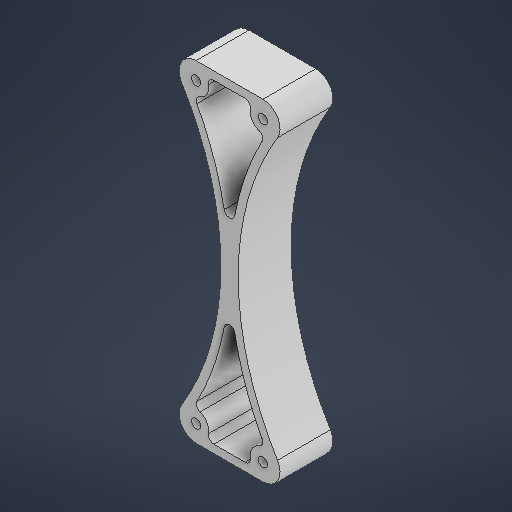
# Autodesk Inventor part: fan_connector_01
Saved by Autodesk Inventor 2026.2 (Build 302298010, 298A)
## iProperties
Created: 2026-05-14
Part Number: fan_connector_01
Material: 一般
Document SubType Name: Modeling
Designer: nyxeon
Density: 1 g/cm^3
Appearance: 既定
Author: nyxeon
Autodesk Inventor part; units mm, degrees
ref_plane "YZ Plane" through (0, 0, 0) normal (1, 0, 0) x (0, 1, 0)
ref_plane "XZ Plane" through (0, 0, 0) normal (0, 1, 0) x (-1, 0, 0)
ref_plane "XY Plane" through (0, 0, 0) normal (0, 0, 1) x (1, 0, 0)
sketch "スケッチ1" plane through (0, 0, 0) normal (0, 0, 1) x (1, 0, 0)
  line L0 (216.819241, 50.161956) -> (211.869241, 50.161956) construction
  line L1 (211.869241, 59.337068) -> (211.869241, 50.161956) construction
  arc A0 (211.869241, 59.337068) -> (211.361116, 60.6691) centre (209.869241, 59.337068) ccw construction
  line L2 (209.369241, 62.9) -> (211.361116, 60.6691) construction
  line L3 (209.369241, 63.9) -> (209.369241, 62.9) construction
  arc A1 (207.869241, 65.4) -> (209.369241, 63.9) centre (209.369241, 65.4) ccw construction
  line L4 (207.869241, 65.4) -> (207.869241, 85.3) construction
  arc A2 (207.869241, 85.3) -> (201.869241, 91.3) centre (201.869241, 85.3) ccw construction
  line L5 (201.869241, 91.3) -> (181.969241, 91.3) construction
  arc A3 (180.469241, 92.8) -> (181.969241, 91.3) centre (181.969241, 92.8) ccw construction
  line L6 (180.469241, 92.8) -> (179.469241, 92.8) construction
  line L7 (179.469241, 92.8) -> (177.238341, 94.791875) construction
  arc A4 (177.238341, 94.791875) -> (175.906309, 95.3) centre (175.906309, 93.3) ccw construction
  line L8 (175.906309, 95.3) -> (154.307286, 95.3) construction
  arc A5 (154.307286, 95.3) -> (137.927787, 100.25) centre (116.569241, 0) ccw construction
  line L9 (95.210695, 100.25) -> (137.927787, 100.25) construction
  arc A6 (95.210695, 100.25) -> (78.831197, 95.3) centre (116.569241, 0) ccw construction
  line L10 (57.232173, 95.3) -> (78.831197, 95.3) construction
  arc A7 (57.232173, 95.3) -> (55.900142, 94.791875) centre (57.232173, 93.3) ccw construction
  line L11 (53.669241, 92.8) -> (55.900142, 94.791875) construction
  line L12 (52.669241, 92.8) -> (53.669241, 92.8) construction
  arc A8 (51.169241, 91.3) -> (52.669241, 92.8) centre (51.169241, 92.8) ccw construction
  line L13 (31.269241, 91.3) -> (51.169241, 91.3) construction
  arc A9 (31.269241, 91.3) -> (25.269241, 85.3) centre (31.269241, 85.3) ccw construction
  line L14 (25.269241, 65.4) -> (25.269241, 85.3) construction
  arc A10 (23.769241, 63.9) -> (25.269241, 65.4) centre (23.769241, 65.4) ccw construction
  line L15 (23.769241, 63.9) -> (23.769241, 62.9) construction
  line L16 (23.769241, 62.9) -> (21.777366, 60.6691) construction
  arc A11 (21.777366, 60.6691) -> (21.269241, 59.337068) centre (23.269241, 59.337068) ccw construction
  line L17 (21.269241, 59.337068) -> (21.269241, 37.738044) construction
  arc A12 (21.269241, 37.738044) -> (16.319241, 21.358546) centre (116.569241, 0) ccw construction
  line L18 (16.319241, -21.358546) -> (16.319241, 21.358546) construction
  arc A13 (16.319241, -21.358546) -> (21.269241, -37.738044) centre (116.569241, 0) ccw construction
  line L19 (21.269241, -59.337068) -> (21.269241, -37.738044) construction
  arc A14 (21.269241, -59.337068) -> (21.777366, -60.6691) centre (23.269241, -59.337068) ccw construction
  line L20 (23.769241, -62.9) -> (21.777366, -60.6691) construction
  line L21 (23.769241, -63.9) -> (23.769241, -62.9) construction
  arc A15 (25.269241, -65.4) -> (23.769241, -63.9) centre (23.769241, -65.4) ccw construction
  line L22 (25.269241, -65.4) -> (25.269241, -85.3) construction
  arc A16 (25.269241, -85.3) -> (31.269241, -91.3) centre (31.269241, -85.3) ccw construction
  line L23 (31.269241, -91.3) -> (51.169241, -91.3) construction
  arc A17 (52.669241, -92.8) -> (51.169241, -91.3) centre (51.169241, -92.8) ccw construction
  line L24 (52.669241, -92.8) -> (53.669241, -92.8) construction
  line L25 (53.669241, -92.8) -> (55.900142, -94.791875) construction
  arc A18 (55.900142, -94.791875) -> (57.232173, -95.3) centre (57.232173, -93.3) ccw construction
  line L26 (57.232173, -95.3) -> (78.831197, -95.3) construction
  arc A19 (78.831197, -95.3) -> (95.210695, -100.25) centre (116.569241, 0) ccw construction
  line L27 (95.210695, -100.25) -> (137.927787, -100.25) construction
  arc A20 (137.927787, -100.25) -> (154.307286, -95.3) centre (116.569241, 0) ccw construction
  line L28 (175.906309, -95.3) -> (154.307286, -95.3) construction
  arc A21 (175.906309, -95.3) -> (177.238341, -94.791875) centre (175.906309, -93.3) ccw construction
  line L29 (179.469241, -92.8) -> (177.238341, -94.791875) construction
  line L30 (180.469241, -92.8) -> (179.469241, -92.8) construction
  arc A22 (181.969241, -91.3) -> (180.469241, -92.8) centre (181.969241, -92.8) ccw construction
  line L31 (201.869241, -91.3) -> (181.969241, -91.3) construction
  arc A23 (201.869241, -91.3) -> (207.869241, -85.3) centre (201.869241, -85.3) ccw construction
  line L32 (207.869241, -65.4) -> (207.869241, -85.3) construction
  arc A24 (209.369241, -63.9) -> (207.869241, -65.4) centre (209.369241, -65.4) ccw construction
  line L33 (209.369241, -63.9) -> (209.369241, -62.9) construction
  line L34 (209.369241, -62.9) -> (211.361116, -60.6691) construction
  arc A25 (211.361116, -60.6691) -> (211.869241, -59.337068) centre (209.869241, -59.337068) ccw construction
  line L35 (211.869241, -59.337068) -> (211.869241, -37.738044) construction
  arc A26 (211.869241, -37.738044) -> (216.819241, -21.358546) centre (116.569241, 0) ccw construction
  line L36 (216.819241, -21.358546) -> (216.819241, 50.161956) construction
  circle A27 centre (31.569241, 85) radius 2.2 construction
  circle A28 centre (39.319241, 77.25) radius 2.2 construction
  circle A29 centre (193.819241, -77.25) radius 2.2 construction
  circle A30 centre (201.569241, -85) radius 2.2 construction
  circle A31 centre (171.569241, -90) radius 2.2 construction
  circle A32 centre (201.581674, -67.012433) radius 1.35 construction
  circle A33 centre (206.569241, -55) radius 2.2 construction
  circle A34 centre (183.581674, 85.012433) radius 1.35 construction
  circle A35 centre (193.819241, 77.25) radius 2.2 construction
  circle A36 centre (201.569241, 85) radius 2.2 construction
  circle A37 centre (171.569241, 90) radius 2.2 construction
  circle A38 centre (201.581674, 67.012433) radius 1.35 construction
  circle A39 centre (206.569241, 55) radius 2.2 construction
  circle A40 centre (183.581674, -85.012433) radius 1.35 construction
  circle A41 centre (26.569241, -55) radius 2.2 construction
  circle A42 centre (31.556808, -67.012433) radius 1.35 construction
  circle A43 centre (61.569241, -90) radius 2.2 construction
  circle A44 centre (31.569241, -85) radius 2.2 construction
  circle A45 centre (61.569241, 90) radius 2.2 construction
  circle A46 centre (31.556808, 67.012433) radius 1.35 construction
  circle A47 centre (26.569241, 55) radius 2.2 construction
  circle A48 centre (49.556808, -85.012433) radius 1.35 construction
  circle A49 centre (49.556808, 85.012433) radius 1.35 construction
  circle A50 centre (39.319241, -77.25) radius 2.2 construction
  arc A51 (50.756956, -72.883353) -> (94.333225, -95.649357) centre (116.569241, 0) ccw construction
  line L37 (50.756956, -72.883353) -> (42.387975, -81.252334) construction
  arc A52 (41.256604, -80.120963) -> (42.387975, -81.252334) centre (41.822289, -80.686649) ccw construction
  line L38 (49.577151, -71.800417) -> (41.256604, -80.120963) construction
  arc A53 (44.768825, -66.99209) -> (49.577151, -71.800417) centre (116.569241, 0) ccw construction
  line L39 (44.768825, -66.99209) -> (36.448278, -75.312637) construction
  arc A54 (35.316907, -74.181266) -> (36.448278, -75.312637) centre (35.882593, -74.746952) ccw construction
  line L40 (43.685888, -65.812285) -> (35.316907, -74.181266) construction
  arc A55 (20.919884, -22.236017) -> (43.685888, -65.812285) centre (116.569241, 0) ccw construction
  line L41 (19.668661, -21) -> (20.919884, -22.236017) construction
  arc A56 (19.668661, 21) -> (19.668661, -21) centre (116.569241, 0) ccw construction
  line L42 (19.668661, 21) -> (20.919884, 22.236017) construction
  arc A57 (43.685888, 65.812285) -> (20.919884, 22.236017) centre (116.569241, 0) ccw construction
  line L43 (43.685888, 65.812285) -> (35.316907, 74.181266) construction
  arc A58 (36.448278, 75.312637) -> (35.316907, 74.181266) centre (35.882593, 74.746952) ccw construction
  line L44 (44.768825, 66.99209) -> (36.448278, 75.312637) construction
  arc A59 (49.577151, 71.800417) -> (44.768825, 66.99209) centre (116.569241, 0) ccw construction
  line L45 (49.577151, 71.800417) -> (41.256604, 80.120963) construction
  arc A60 (42.387975, 81.252334) -> (41.256604, 80.120963) centre (41.822289, 80.686649) ccw construction
  line L46 (50.756956, 72.883353) -> (42.387975, 81.252334) construction
  arc A61 (94.333225, 95.649357) -> (50.756956, 72.883353) centre (116.569241, 0) ccw construction
  line L47 (95.569241, 96.90058) -> (94.333225, 95.649357) construction
  arc A62 (137.569241, 96.90058) -> (95.569241, 96.90058) centre (116.569241, 0) ccw construction
  line L48 (137.569241, 96.90058) -> (138.805258, 95.649357) construction
  arc A63 (182.381526, 72.883353) -> (138.805258, 95.649357) centre (116.569241, 0) ccw construction
  line L49 (182.381526, 72.883353) -> (190.750507, 81.252334) construction
  arc A64 (191.881878, 80.120963) -> (190.750507, 81.252334) centre (191.316193, 80.686649) ccw construction
  line L50 (183.561332, 71.800417) -> (191.881878, 80.120963) construction
  arc A65 (188.369658, 66.99209) -> (183.561332, 71.800417) centre (116.569241, 0) ccw construction
  line L51 (188.369658, 66.99209) -> (196.690204, 75.312637) construction
  arc A66 (197.821575, 74.181266) -> (196.690204, 75.312637) centre (197.25589, 74.746952) ccw construction
  line L52 (189.452594, 65.812285) -> (197.821575, 74.181266) construction
  arc A67 (212.218599, 22.236017) -> (189.452594, 65.812285) centre (116.569241, 0) ccw construction
  line L53 (213.469822, 21) -> (212.218599, 22.236017) construction
  arc A68 (213.469822, -21) -> (213.469822, 21) centre (116.569241, 0) ccw construction
  line L54 (213.469822, -21) -> (212.218599, -22.236017) construction
  arc A69 (189.452594, -65.812285) -> (212.218599, -22.236017) centre (116.569241, 0) ccw construction
  line L55 (189.452594, -65.812285) -> (197.821575, -74.181266) construction
  arc A70 (196.690204, -75.312637) -> (197.821575, -74.181266) centre (197.25589, -74.746952) ccw construction
  line L56 (188.369658, -66.99209) -> (196.690204, -75.312637) construction
  arc A71 (183.561332, -71.800417) -> (188.369658, -66.99209) centre (116.569241, 0) ccw construction
  line L57 (183.561332, -71.800417) -> (191.881878, -80.120963) construction
  arc A72 (190.750507, -81.252334) -> (191.881878, -80.120963) centre (191.316193, -80.686649) ccw construction
  line L58 (182.381526, -72.883353) -> (190.750507, -81.252334) construction
  arc A73 (138.805258, -95.649357) -> (182.381526, -72.883353) centre (116.569241, 0) ccw construction
  line L59 (137.569241, -96.90058) -> (138.805258, -95.649357) construction
  arc A74 (95.569241, -96.90058) -> (137.569241, -96.90058) centre (116.569241, 0) ccw construction
  line L60 (95.569241, -96.90058) -> (94.333225, -95.649357) construction
  line L61 (12.069241, 50.161956) -> (7.119241, 50.161956) construction
  line L62 (7.119241, 59.337068) -> (7.119241, 50.161956) construction
  arc A75 (7.119241, 59.337068) -> (6.611116, 60.6691) centre (5.119241, 59.337068) ccw construction
  line L63 (4.619241, 62.9) -> (6.611116, 60.6691) construction
  line L64 (4.619241, 63.9) -> (4.619241, 62.9) construction
  arc A76 (3.119241, 65.4) -> (4.619241, 63.9) centre (4.619241, 65.4) ccw construction
  line L65 (3.119241, 65.4) -> (3.119241, 85.3) construction
  arc A77 (3.119241, 85.3) -> (-2.880759, 91.3) centre (-2.880759, 85.3) ccw construction
  line L66 (-2.880759, 91.3) -> (-22.780759, 91.3) construction
  arc A78 (-24.280759, 92.8) -> (-22.780759, 91.3) centre (-22.780759, 92.8) ccw construction
  line L67 (-24.280759, 92.8) -> (-25.280759, 92.8) construction
  line L68 (-25.280759, 92.8) -> (-27.511659, 94.791875) construction
  arc A79 (-27.511659, 94.791875) -> (-28.843691, 95.3) centre (-28.843691, 93.3) ccw construction
  line L69 (-28.843691, 95.3) -> (-50.442714, 95.3) construction
  arc A80 (-50.442714, 95.3) -> (-66.822213, 100.25) centre (-88.180759, 0) ccw construction
  line L70 (-109.539305, 100.25) -> (-66.822213, 100.25) construction
  arc A81 (-109.539305, 100.25) -> (-125.918803, 95.3) centre (-88.180759, 0) ccw construction
  line L71 (-147.517827, 95.3) -> (-125.918803, 95.3) construction
  arc A82 (-147.517827, 95.3) -> (-148.849858, 94.791875) centre (-147.517827, 93.3) ccw construction
  line L72 (-151.080759, 92.8) -> (-148.849858, 94.791875) construction
  line L73 (-152.080759, 92.8) -> (-151.080759, 92.8) construction
  arc A83 (-153.580759, 91.3) -> (-152.080759, 92.8) centre (-153.580759, 92.8) ccw construction
  line L74 (-173.480759, 91.3) -> (-153.580759, 91.3) construction
  arc A84 (-173.480759, 91.3) -> (-179.480759, 85.3) centre (-173.480759, 85.3) ccw construction
  line L75 (-179.480759, 65.4) -> (-179.480759, 85.3) construction
  arc A85 (-180.980759, 63.9) -> (-179.480759, 65.4) centre (-180.980759, 65.4) ccw construction
  line L76 (-180.980759, 63.9) -> (-180.980759, 62.9) construction
  line L77 (-180.980759, 62.9) -> (-182.972634, 60.6691) construction
  arc A86 (-182.972634, 60.6691) -> (-183.480759, 59.337068) centre (-181.480759, 59.337068) ccw construction
  line L78 (-183.480759, 59.337068) -> (-183.480759, 37.738044) construction
  arc A87 (-183.480759, 37.738044) -> (-188.430759, 21.358546) centre (-88.180759, 0) ccw construction
  line L79 (-188.430759, -21.358546) -> (-188.430759, 21.358546) construction
  arc A88 (-188.430759, -21.358546) -> (-183.480759, -37.738044) centre (-88.180759, 0) ccw construction
  line L80 (-183.480759, -59.337068) -> (-183.480759, -37.738044) construction
  arc A89 (-183.480759, -59.337068) -> (-182.972634, -60.6691) centre (-181.480759, -59.337068) ccw construction
  line L81 (-180.980759, -62.9) -> (-182.972634, -60.6691) construction
  line L82 (-180.980759, -63.9) -> (-180.980759, -62.9) construction
  arc A90 (-179.480759, -65.4) -> (-180.980759, -63.9) centre (-180.980759, -65.4) ccw construction
  line L83 (-179.480759, -65.4) -> (-179.480759, -85.3) construction
  arc A91 (-179.480759, -85.3) -> (-173.480759, -91.3) centre (-173.480759, -85.3) ccw construction
  line L84 (-173.480759, -91.3) -> (-153.580759, -91.3) construction
  arc A92 (-152.080759, -92.8) -> (-153.580759, -91.3) centre (-153.580759, -92.8) ccw construction
  line L85 (-152.080759, -92.8) -> (-151.080759, -92.8) construction
  line L86 (-151.080759, -92.8) -> (-148.849858, -94.791875) construction
  arc A93 (-148.849858, -94.791875) -> (-147.517827, -95.3) centre (-147.517827, -93.3) ccw construction
  line L87 (-147.517827, -95.3) -> (-125.918803, -95.3) construction
  arc A94 (-125.918803, -95.3) -> (-109.539305, -100.25) centre (-88.180759, 0) ccw construction
  line L88 (-109.539305, -100.25) -> (-66.822213, -100.25) construction
  arc A95 (-66.822213, -100.25) -> (-50.442714, -95.3) centre (-88.180759, 0) ccw construction
  line L89 (-28.843691, -95.3) -> (-50.442714, -95.3) construction
  arc A96 (-28.843691, -95.3) -> (-27.511659, -94.791875) centre (-28.843691, -93.3) ccw construction
  line L90 (-25.280759, -92.8) -> (-27.511659, -94.791875) construction
  line L91 (-24.280759, -92.8) -> (-25.280759, -92.8) construction
  arc A97 (-22.780759, -91.3) -> (-24.280759, -92.8) centre (-22.780759, -92.8) ccw construction
  line L92 (-2.880759, -91.3) -> (-22.780759, -91.3) construction
  arc A98 (-2.880759, -91.3) -> (3.119241, -85.3) centre (-2.880759, -85.3) ccw construction
  line L93 (3.119241, -65.4) -> (3.119241, -85.3) construction
  arc A99 (4.619241, -63.9) -> (3.119241, -65.4) centre (4.619241, -65.4) ccw construction
  line L94 (4.619241, -63.9) -> (4.619241, -62.9) construction
  line L95 (4.619241, -62.9) -> (6.611116, -60.6691) construction
  arc A100 (6.611116, -60.6691) -> (7.119241, -59.337068) centre (5.119241, -59.337068) ccw construction
  line L96 (7.119241, -59.337068) -> (7.119241, -37.738044) construction
  arc A101 (7.119241, -37.738044) -> (12.069241, -21.358546) centre (-88.180759, 0) ccw construction
  line L97 (12.069241, -21.358546) -> (12.069241, 50.161956) construction
  circle A102 centre (-173.180759, 85) radius 2.2 construction
  circle A103 centre (-165.430759, 77.25) radius 2.2 construction
  circle A104 centre (-10.930759, -77.25) radius 2.2 construction
  circle A105 centre (-3.180759, -85) radius 2.2 construction
  circle A106 centre (-33.180759, -90) radius 2.2 construction
  circle A107 centre (-3.168326, -67.012433) radius 1.35 construction
  circle A108 centre (1.819241, -55) radius 2.2 construction
  circle A109 centre (-21.168326, 85.012433) radius 1.35 construction
  circle A110 centre (-10.930759, 77.25) radius 2.2 construction
  circle A111 centre (-3.180759, 85) radius 2.2 construction
  circle A112 centre (-33.180759, 90) radius 2.2 construction
  circle A113 centre (-3.168326, 67.012433) radius 1.35 construction
  circle A114 centre (1.819241, 55) radius 2.2 construction
  circle A115 centre (-21.168326, -85.012433) radius 1.35 construction
  circle A116 centre (-178.180759, -55) radius 2.2 construction
  circle A117 centre (-173.193192, -67.012433) radius 1.35 construction
  circle A118 centre (-143.180759, -90) radius 2.2 construction
  circle A119 centre (-173.180759, -85) radius 2.2 construction
  circle A120 centre (-143.180759, 90) radius 2.2 construction
  circle A121 centre (-173.193192, 67.012433) radius 1.35 construction
  circle A122 centre (-178.180759, 55) radius 2.2 construction
  circle A123 centre (-155.193192, -85.012433) radius 1.35 construction
  circle A124 centre (-155.193192, 85.012433) radius 1.35 construction
  circle A125 centre (-165.430759, -77.25) radius 2.2 construction
  arc A126 (-153.993044, -72.883353) -> (-110.416775, -95.649357) centre (-88.180759, 0) ccw construction
  line L98 (-153.993044, -72.883353) -> (-162.362025, -81.252334) construction
  arc A127 (-163.493396, -80.120963) -> (-162.362025, -81.252334) centre (-162.927711, -80.686649) ccw construction
  line L99 (-155.172849, -71.800417) -> (-163.493396, -80.120963) construction
  arc A128 (-159.981175, -66.99209) -> (-155.172849, -71.800417) centre (-88.180759, 0) ccw construction
  line L100 (-159.981175, -66.99209) -> (-168.301722, -75.312637) construction
  arc A129 (-169.433093, -74.181266) -> (-168.301722, -75.312637) centre (-168.867407, -74.746952) ccw construction
  line L101 (-161.064112, -65.812285) -> (-169.433093, -74.181266) construction
  arc A130 (-183.830116, -22.236017) -> (-161.064112, -65.812285) centre (-88.180759, 0) ccw construction
  line L102 (-185.081339, -21) -> (-183.830116, -22.236017) construction
  arc A131 (-185.081339, 21) -> (-185.081339, -21) centre (-88.180759, 0) ccw construction
  line L103 (-185.081339, 21) -> (-183.830116, 22.236017) construction
  arc A132 (-161.064112, 65.812285) -> (-183.830116, 22.236017) centre (-88.180759, 0) ccw construction
  line L104 (-161.064112, 65.812285) -> (-169.433093, 74.181266) construction
  arc A133 (-168.301722, 75.312637) -> (-169.433093, 74.181266) centre (-168.867407, 74.746952) ccw construction
  line L105 (-159.981175, 66.99209) -> (-168.301722, 75.312637) construction
  arc A134 (-155.172849, 71.800417) -> (-159.981175, 66.99209) centre (-88.180759, 0) ccw construction
  line L106 (-155.172849, 71.800417) -> (-163.493396, 80.120963) construction
  arc A135 (-162.362025, 81.252334) -> (-163.493396, 80.120963) centre (-162.927711, 80.686649) ccw construction
  line L107 (-153.993044, 72.883353) -> (-162.362025, 81.252334) construction
  arc A136 (-110.416775, 95.649357) -> (-153.993044, 72.883353) centre (-88.180759, 0) ccw construction
  line L108 (-109.180759, 96.90058) -> (-110.416775, 95.649357) construction
  arc A137 (-67.180759, 96.90058) -> (-109.180759, 96.90058) centre (-88.180759, 0) ccw construction
  line L109 (-67.180759, 96.90058) -> (-65.944742, 95.649357) construction
  arc A138 (-22.368474, 72.883353) -> (-65.944742, 95.649357) centre (-88.180759, 0) ccw construction
  line L110 (-22.368474, 72.883353) -> (-13.999493, 81.252334) construction
  arc A139 (-12.868122, 80.120963) -> (-13.999493, 81.252334) centre (-13.433807, 80.686649) ccw construction
  line L111 (-21.188668, 71.800417) -> (-12.868122, 80.120963) construction
  arc A140 (-16.380342, 66.99209) -> (-21.188668, 71.800417) centre (-88.180759, 0) ccw construction
  line L112 (-16.380342, 66.99209) -> (-8.059796, 75.312637) construction
  arc A141 (-6.928425, 74.181266) -> (-8.059796, 75.312637) centre (-7.49411, 74.746952) ccw construction
  line L113 (-15.297406, 65.812285) -> (-6.928425, 74.181266) construction
  arc A142 (7.468599, 22.236017) -> (-15.297406, 65.812285) centre (-88.180759, 0) ccw construction
  line L114 (8.719822, 21) -> (7.468599, 22.236017) construction
  arc A143 (8.719822, -21) -> (8.719822, 21) centre (-88.180759, 0) ccw construction
  line L115 (8.719822, -21) -> (7.468599, -22.236017) construction
  arc A144 (-15.297406, -65.812285) -> (7.468599, -22.236017) centre (-88.180759, 0) ccw construction
  line L116 (-15.297406, -65.812285) -> (-6.928425, -74.181266) construction
  arc A145 (-8.059796, -75.312637) -> (-6.928425, -74.181266) centre (-7.49411, -74.746952) ccw construction
  line L117 (-16.380342, -66.99209) -> (-8.059796, -75.312637) construction
  arc A146 (-21.188668, -71.800417) -> (-16.380342, -66.99209) centre (-88.180759, 0) ccw construction
  line L118 (-21.188668, -71.800417) -> (-12.868122, -80.120963) construction
  arc A147 (-13.999493, -81.252334) -> (-12.868122, -80.120963) centre (-13.433807, -80.686649) ccw construction
  line L119 (-22.368474, -72.883353) -> (-13.999493, -81.252334) construction
  arc A148 (-65.944742, -95.649357) -> (-22.368474, -72.883353) centre (-88.180759, 0) ccw construction
  line L120 (-67.180759, -96.90058) -> (-65.944742, -95.649357) construction
  arc A149 (-109.180759, -96.90058) -> (-67.180759, -96.90058) centre (-88.180759, 0) ccw construction
  line L121 (-109.180759, -96.90058) -> (-110.416775, -95.649357) construction
  arc A150 (-14.801793, -66.307898) -> (8.393365, -21.322489) centre (-88.180759, 0) ccw construction
  arc A151 (18.995117, -21.322489) -> (42.190275, -66.307898) centre (116.569241, 0) ccw construction
  line L122 (-88.180759, 0) -> (116.569241, 0) construction
  circle A152 centre (1.819241, -55) radius 6.325116 construction
  circle A153 centre (26.569241, -55) radius 6.325116 construction
  arc A154 (19.668661, -21) -> (95.569241, -96.90058) centre (116.569241, 0) ccw construction
  circle A155 centre (1.819241, 55) radius 6.325116 construction
  circle A156 centre (26.569241, 55) radius 6.325116 construction
  line L123 (26.569241, -55) -> (116.569241, 0) construction
  arc A157 (31.966347, 51.701768) -> (31.966347, -51.701768) centre (116.569241, 0) ccw
  arc A158 (-3.577865, -51.701768) -> (-3.577865, 51.701768) centre (-88.180759, 0) ccw
  arc A159 (26.569241, -61.325116) -> (31.966347, -51.701768) centre (26.569241, -55) ccw
  arc A160 (-3.577865, -51.701768) -> (1.819241, -61.325116) centre (1.819241, -55) ccw
  arc A161 (1.819241, 61.325116) -> (-3.577865, 51.701768) centre (1.819241, 55) ccw
  arc A162 (31.966347, 51.701768) -> (26.569241, 61.325116) centre (26.569241, 55) ccw
  line L124 (1.819241, -61.325116) -> (26.569241, -61.325116)
  line L125 (1.819241, 61.325116) -> (26.569241, 61.325116)
  circle A163 centre (1.819241, -55) radius 1.7
  circle A164 centre (26.569241, -55) radius 1.7
  circle A165 centre (26.569241, 55) radius 1.7
  circle A166 centre (1.819241, 55) radius 1.7
  point P0 (0, 0)
  dimension "d0" = 12.65023
  dimension "d1" = 3.4
  constraints: 24 point on circle, 15 centre point, 15 coincident, 8 end point, 5 equal radius, 3 concentric, 2 horizontal, 2 tangent, 1 horizontal alignment, 1 parallel, 1 point on line, 1 vertical alignment, 16 other
  measures "d0" diameter of A152
  measures "d1" diameter of A163
extrude "押し出し1" add sketch "スケッチ1" along normal blind 15.8 and the other way blind 3.8
shell "シェル1" thickness 3 removed faces 1 at (17.895085, -44.391215, 15.8)
sketch "スケッチ3" plane through (0, 0, 15.8) normal (0, 0, 1) x (1, 0, 0)
  arc A0 (0.641705, -50.4499) -> (0.641705, 50.4499) centre (-88.180759, 0) ccw
  arc A1 (27.746777, 50.4499) -> (27.746777, -50.4499) centre (116.569241, 0) ccw
  line L0 (13.958227, 1.5) -> (14.430255, 1.5)
  line L1 (13.958227, -1.5) -> (14.430255, -1.5)
  point P0 (0, 0)
  dimension "d10" = 3
  constraints: 4 end point, 4 point on circle, 2 parallel, 1 horizontal
  measures "d10" distance between parallel lines of L1 L0
extrude "押し出し3" add sketch "スケッチ3" against normal up to surface (16.6 mm away)
fillet "フィレット1" radius 2 12 edges at (5.1409, -58.3251, 7.5) (0.6417, -50.4499, 7.5) (23.2476, -58.3251, 7.5) (27.7468, -50.4499, 7.5) (27.7468, 50.4499, 7.5) (23.2476, 58.3251, 7.5) (0.6417, 50.4499, 7.5) (5.1409, 58.3251, 7.5) (13.9582, -1.5, 7.5) (14.4303, -1.5, 7.5) (13.9582, 1.5, 7.5) (14.4303, 1.5, 7.5)
sketch "スケッチ4" plane through (8.386894, 58.325116, -0.8) normal (0, 0, 1) x (1, 0, 0)
  arc A0 (3.841432, -39.546456) -> (7.773261, -39.546456) centre (5.807347, -39.178788) ccw
  arc A1 (17.854599, -10.6227) -> (7.773261, -39.546456) centre (108.182347, -58.325116) ccw
  arc A2 (17.854599, -10.6227) -> (16.711822, -7.789145) centre (16.086067, -9.688732) ccw
  arc A3 (13.575187, -2.395557) -> (16.711822, -7.789145) centre (18.182347, -3.325116) ccw
  arc A4 (13.575187, -2.395557) -> (11.614694, 0) centre (11.614694, -2) ccw
  line L0 (0, 0) -> (11.614694, 0)
  arc A5 (0, 0) -> (-1.960493, -2.395557) centre (0, -2) ccw
  arc A6 (-5.097129, -7.789145) -> (-1.960493, -2.395557) centre (-6.567653, -3.325116) ccw
  arc A7 (-5.097129, -7.789145) -> (-6.239905, -10.6227) centre (-4.471374, -9.688732) ccw
  arc A8 (3.841432, -39.546456) -> (-6.239905, -10.6227) centre (-96.567653, -58.325116) ccw
  arc A9 (7.773261, -77.103775) -> (3.841432, -77.103775) centre (5.807347, -77.471444) ccw
  arc A10 (-6.239905, -106.027531) -> (3.841432, -77.103775) centre (-96.567653, -58.325116) ccw
  arc A11 (-6.239905, -106.027531) -> (-5.097129, -108.861086) centre (-4.471374, -106.961499) ccw
  arc A12 (-1.960493, -114.254674) -> (-5.097129, -108.861086) centre (-6.567653, -113.325116) ccw
  arc A13 (-1.960493, -114.254674) -> (0, -116.650231) centre (0, -114.650231) ccw
  line L1 (11.614694, -116.650231) -> (0, -116.650231)
  arc A14 (11.614694, -116.650231) -> (13.575187, -114.254674) centre (11.614694, -114.650231) ccw
  arc A15 (16.711822, -108.861086) -> (13.575187, -114.254674) centre (18.182347, -113.325116) ccw
  arc A16 (16.711822, -108.861086) -> (17.854599, -106.027531) centre (16.086067, -106.961499) ccw
  arc A17 (7.773261, -77.103775) -> (17.854599, -106.027531) centre (108.182347, -58.325116) ccw
  point P0 (-8.386894, -58.325116)
extrude "押し出し4" cut sketch "スケッチ4" against normal blind 1
